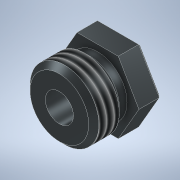
# Autodesk Inventor part: 3-锁紧螺母
Saved by Autodesk Inventor 2022 (Build 260153000, 153)
## iProperties
Created: 2023-01-24
Part Number: 3-锁紧螺母
Material: 灰口铁
Document SubType Name: Modeling
Designer: Lzy18
Density: 7.15 g/cm^3
Appearance: 灰口铁
Author: Lzy18
Autodesk Inventor part; units mm, degrees
ref_plane "YZ Plane" through (0, 0, 0) normal (1, 0, 0) x (0, 1, 0)
ref_plane "XZ Plane" through (0, 0, 0) normal (0, 1, 0) x (-1, 0, 0)
ref_plane "XY Plane" through (0, 0, 0) normal (0, 0, 1) x (1, 0, 0)
sketch "草图1" plane through (0, 0, 0) normal (0, 0, 1) x (1, 0, 0)
  line L0 (8.0829, 14) -> (16.1658, 0)
  line L1 (16.1658, 0) -> (8.0829, -14)
  line L2 (8.0829, -14) -> (-8.0829, -14)
  line L3 (-8.0829, -14) -> (-16.1658, 0)
  line L4 (-16.1658, 0) -> (-8.0829, 14)
  line L5 (-8.0829, 14) -> (8.0829, 14)
  point P0 (0, 0)
  point P1 (0, 0)
  constraints: 12 end point, 13 other
extrude "拉伸1" add sketch "草图1" along normal blind 9
sketch "草图2" plane through (0, 0, 9) normal (0, 0, 1) x (1, 0, 0)
  circle A0 centre (0, 0) radius 11.5
  dimension "d4" = 23
  constraints: 1 centre point, 1 coincident
  measures "d4" diameter of A0
extrude "拉伸2" add sketch "草图2" along normal blind 3
sketch "草图3" plane through (0, 0, 12) normal (0, 0, 1) x (1, 0, 0)
  circle A0 centre (0, 0) radius 13.5
  dimension "d7" = 27
  constraints: 1 centre point, 1 coincident
  measures "d7" diameter of A0
extrude "拉伸3" add sketch "草图3" along normal blind 12
chamfer "倒角1" distance 2 angle 45 2 edges at (-13.5, 0, 24) (-13.5, 0, 12)
sketch "草图4" plane through (0, 0, 24) normal (0, 0, 1) x (1, 0, 0)
  circle A0 centre (0, 0) radius 11.5 projected
  constraints: 1 coincident
hole "孔1" at (0, 0, 24) direction (0, 0, -1) diameter 11 end through all
thread "螺纹1" size "M27x3" designation "M27" class "6g" standard "GB Metric profile" length 48
chamfer "倒角2" distance 1 angle 45 6 edges at (12.1244, -7, 0) (12.1244, 7, 0) (0, 14, 0) (-12.1244, 7, 0) (0, -14, 0) (-12.1244, -7, 0)
